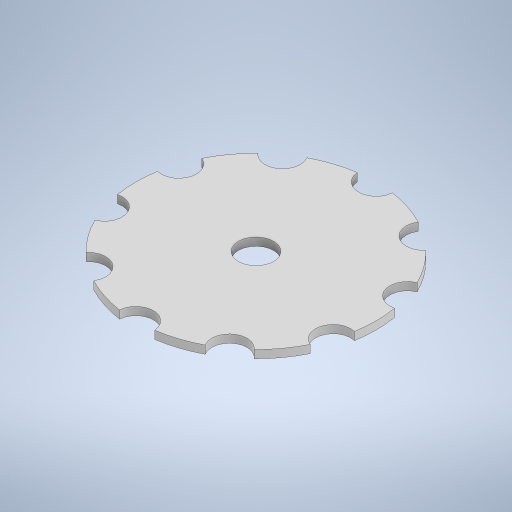
# Autodesk Inventor part: M15_10
Saved by Autodesk Inventor 2024.1 (Build 281209000, 209)
## iProperties
Created: 2024-03-26
Part Number: M15_10
Material: 一般
Document SubType Name: Modeling
Designer: hibik
Density: 1 g/cm^3
Appearance: 既定
Author: hibik
Autodesk Inventor part; units mm, degrees
ref_plane "YZ Plane" through (0, 0, 0) normal (1, 0, 0) x (0, 1, 0)
ref_plane "XZ Plane" through (0, 0, 0) normal (0, 1, 0) x (-1, 0, 0)
ref_plane "XY Plane" through (0, 0, 0) normal (0, 0, 1) x (1, 0, 0)
sketch "スケッチ1" plane through (0, 0, 0) normal (0, 1, 0) x (-1, 0, 0)
  circle A0 centre (0, 0) radius 75 construction
  circle A1 centre (0, 0) radius 56.25 construction
  circle A2 centre (0, 0) radius 90 construction
  line L0 (89.2264, 11.775) -> (49.8187, 26.1182)
  line L1 (89.2264, -11.775) -> (49.8187, -26.1182)
  line L2 (126, 0) -> (-126, 0) projected
  line L3 (89.2264, 11.775) -> (89.2264, -11.775)
  line L4 (65.2645, 61.9721) -> (24.9522, 50.4128)
  line L5 (79.1068, 42.9198) -> (55.6561, 8.1526)
  line L6 (65.2645, 61.9721) -> (79.1068, 42.9198)
  line L7 (16.3738, 88.498) -> (-9.4451, 55.4514)
  line L8 (38.7712, 81.2207) -> (40.2347, 39.3094)
  line L9 (16.3738, 88.498) -> (38.7712, 81.2207)
  line L10 (-38.7712, 81.2207) -> (-40.2347, 39.3094)
  line L11 (-16.3738, 88.498) -> (9.4451, 55.4514)
  line L12 (-38.7712, 81.2207) -> (-16.3738, 88.498)
  line L13 (-79.1068, 42.9198) -> (-55.6561, 8.1526)
  line L14 (-65.2645, 61.9721) -> (-24.9522, 50.4128)
  line L15 (-79.1068, 42.9198) -> (-65.2645, 61.9721)
  line L16 (-89.2264, -11.775) -> (-49.8187, -26.1182)
  line L17 (-89.2264, 11.775) -> (-49.8187, 26.1182)
  line L18 (-89.2264, -11.775) -> (-89.2264, 11.775)
  line L19 (-65.2645, -61.9721) -> (-24.9522, -50.4128)
  line L20 (-79.1068, -42.9198) -> (-55.6561, -8.1526)
  line L21 (-65.2645, -61.9721) -> (-79.1068, -42.9198)
  line L22 (-16.3738, -88.498) -> (9.4451, -55.4514)
  line L23 (-38.7712, -81.2207) -> (-40.2347, -39.3094)
  line L24 (-16.3738, -88.498) -> (-38.7712, -81.2207)
  line L25 (38.7712, -81.2207) -> (40.2347, -39.3094)
  line L26 (16.3738, -88.498) -> (-9.4451, -55.4514)
  line L27 (38.7712, -81.2207) -> (16.3738, -88.498)
  line L28 (79.1068, -42.9198) -> (55.6561, -8.1526)
  line L29 (65.2645, -61.9721) -> (24.9522, -50.4128)
  line L30 (79.1068, -42.9198) -> (65.2645, -61.9721)
  line L31 (72.8751, -17.7264) -> (69.3765, -28.4939) construction
  circle A3 centre (71.3292, -23.1763) radius 11
  line L32 (73.1573, -12.3292) -> (0, 0) construction
  line L33 (0, 0) -> (66.4324, -33.0262) construction
  line L34 (71.3292, -23.1763) -> (0, 0) construction
  circle A4 centre (71.3292, 23.1763) radius 11
  circle A5 centre (44.0839, 60.6763) radius 11
  circle A6 centre (0, 75) radius 11
  circle A7 centre (-44.0839, 60.6763) radius 11
  circle A8 centre (-71.3292, 23.1763) radius 11
  circle A9 centre (-71.3292, -23.1763) radius 11
  circle A10 centre (-44.0839, -60.6763) radius 11
  circle A11 centre (0, -75) radius 11
  circle A12 centre (44.0839, -60.6763) radius 11
  circle A13 centre (0, 0) radius 75
  circle A14 centre (0, 0) radius 11
  point P0 (71.1258, -23.1102)
  point P1 (66.4324, 33.0262)
  point P2 (73.1573, 12.3292)
  point P3 (34.3326, 65.7668)
  point P4 (51.9386, 52.9753)
  point P5 (-10.881, 73.3867)
  point P6 (10.881, 73.3867)
  point P7 (-51.9386, 52.9753)
  point P8 (-34.3326, 65.7668)
  point P9 (-73.1573, 12.3292)
  point P10 (-66.4324, 33.0262)
  point P11 (-66.4324, -33.0262)
  point P12 (-73.1573, -12.3292)
  point P13 (-34.3326, -65.7668)
  point P14 (-51.9386, -52.9753)
  point P15 (10.881, -73.3867)
  point P16 (-10.881, -73.3867)
  point P17 (51.9386, -52.9753)
  point P18 (34.3326, -65.7668)
  point P19 (73.9521, 12.4935)
  point P20 (67.172, 33.3605)
  point P21 (52.485, 53.5754)
  point P22 (34.7345, 66.4719)
  point P23 (10.9704, 74.1933)
  point P24 (-10.9704, 74.1933)
  point P25 (-34.7345, 66.4719)
  point P26 (-52.485, 53.5754)
  point P27 (-67.172, 33.3605)
  point P28 (-73.9521, 12.4935)
  point P29 (-73.9521, -12.4935)
  point P30 (-67.172, -33.3605)
  point P31 (-52.485, -53.5754)
  point P32 (-34.7345, -66.4719)
  point P33 (-10.9704, -74.1933)
  point P34 (10.9704, -74.1933)
  point P35 (34.7345, -66.4719)
  point P36 (52.485, -53.5754)
  point P37 (67.172, -33.3605)
  point P38 (73.9521, -12.4935)
  dimension "d0" = 150
  dimension "d1" = 112.5
  dimension "d2" = 180
  dimension "d3" = 20
  dimension "d4" = 20
  dimension "d5" = 23.55
  dimension "d17" = 360
  dimension "d19" = 22
  dimension "d22" = 360
  dimension "d26" = 22
  constraints: 68 end point, 27 point on circle, 15 centre point, 6 coincident, 3 point on line, 2 tangent, 1 concentric, 1 midpoint, 1 vertical, 112 other
  measures "d0" diameter of A0
  measures "d1" diameter of A1
  measures "d2" diameter of A2
  measures "d3" angle of L2 L0
  measures "d4" angle of L1 L2
  measures "d5" distance of L0.start L1.start
  measures "d19" diameter of A3
  measures "d26" diameter of A14
extrude "押し出し2" add sketch "スケッチ1" along normal blind 5 contours A13 L2 A14 A8 A7 A6 A5 A4 | A13 A3 A12 A11 A10 A9 L2 A14
equation "\"d4\" = d3"
